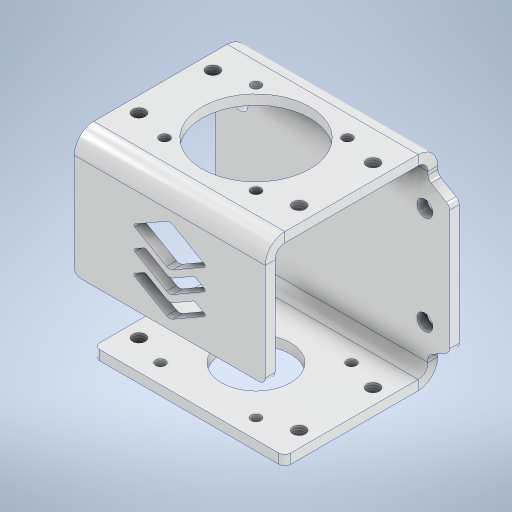
# Autodesk Inventor part: Z-Axis Drive Mount
Saved by Autodesk Inventor 2024 (Build 280153000, 153)
## iProperties
Created: 2024-12-16
Part Number: Z-Axis Drive Mount
Material: Aluminum 6061
Document SubType Name: Sheet Metal
Designer: Ishaan
Density: 2.7 g/cm^3
Sheet Metal Rule: SendCutSend_1-8_Alu
Appearance: Aluminum - Flat
Flat Pattern Width: 7.6 cm
Flat Pattern Length: 19.5495 cm
Flat Pattern Area: 148.576 cm^2
Sheet Metal Width: 76.000 mm
Sheet Metal Length: 195.495 mm
Sheet Metal Area: 14857.623 mm^2
Author: Ishaan
Autodesk Inventor part; units mm, degrees
note: some values were not read from the file. Chosen so that the rebuilt part matches the saved one: direction of "Hole1"; direction of "Hole2"; direction of "Hole3"; direction of "Hole4".
ref_plane "YZ Plane" through (0, 0, 0) normal (1, 0, 0) x (0, 1, 0)
ref_plane "XZ Plane" through (0, 0, 0) normal (0, 1, 0) x (-1, 0, 0)
ref_plane "XY Plane" through (0, 0, 0) normal (0, 0, 1) x (1, 0, 0)
sketch "Sketch1" plane through (0, 0, 0) normal (0, 0, 1) x (1, 0, 0)
  line L0 (31, -30.025) -> (-31, -30.025)
  line L1 (-31, -30.025) -> (-31, 30.025)
  line L2 (-31, 30.025) -> (31, 30.025)
  line L3 (31, 30.025) -> (31, -30.025)
  line L4 (31, -30.025) -> (-31, 30.025) construction
  line L5 (-31, -30.025) -> (31, 30.025) construction
  point P0 (0, 0)
  dimension "d0" = 62
  dimension "d1" = 60.05
  measures "d0" distance of L1.end L2.end
  measures "d1" distance of L0.end L1.end
extrude "Plate1" add sketch "Sketch1" along normal blind 3.175
sketch "Sketch2" plane through (-31, 30.025, 3.175) normal (0, 1, 0) x (-1, 0, 0)
  line L0 (-62, 0) -> (0, 0)
  line L1 (0, 0) -> (0, 71.825)
  line L2 (0, 71.825) -> (-62, 71.825)
  line L3 (-62, 71.825) -> (-62, 0)
  constraints: 6 end point, 1 horizontal, 1 perpendicular, 1 vertical
edge flange "Flange1" height 75 angle 90 thickness 3.175 bend radius 3.175 thickness toward (0, 1, 0) relief tear relief width 3.175 relief depth 1.5875 edges at (0, 30.025, 3.175) wall of the first edge with corners at (31, 30.025, 3.175) (-31, 30.025, 3.175) (-31, 30.025, 75) (31, 30.025, 75)
bend "Bend1"
corner "Corner1"
sketch "Sketch3" plane through (31, -30.025, 3.175) normal (0, -1, 0) x (1, 0, 0)
  line L0 (-62, 0) -> (0, 0)
  line L1 (0, 0) -> (0, 71.825)
  line L2 (0, 71.825) -> (-62, 71.825)
  line L3 (-62, 71.825) -> (-62, 0)
  constraints: 6 end point, 1 horizontal, 1 perpendicular, 1 vertical
edge flange "Flange2" height 75 angle 90 thickness 3.175 bend radius 3.175 thickness toward (0, -1, 0) relief tear relief width 3.175 relief depth 1.5875 edges at (0, -30.025, 3.175) wall of the first edge with corners at (-31, -30.025, 3.175) (31, -30.025, 3.175) (31, -30.025, 75) (-31, -30.025, 75)
bend "Bend2"
corner "Corner2"
sketch "Sketch4" plane through (-31, 33.2, 75) normal (0, 1, 0) x (1, 0, 0)
  line L0 (52, 26) -> (10, 26) construction
  line L1 (10, 26) -> (10, 68) construction
  line L2 (10, 68) -> (52, 68) construction
  line L3 (52, 68) -> (52, 26) construction
  line L4 (52, 26) -> (10, 68) construction
  line L5 (10, 26) -> (52, 68) construction
  circle A0 centre (31, 47) radius 21 construction
  line L6 (0, 0) -> (0, 68.65) projected
  line L7 (0, 25.35) -> (62, 25.35)
  line L8 (62, 68.65) -> (0, 68.65) projected
  line L9 (0, 0) -> (0, 68.65) projected
  line L10 (62, 0) -> (0, 0) projected
  line L11 (62, 68.65) -> (62, 0) projected
  line L12 (62, 68.65) -> (62, 0) projected
  circle A1 centre (31, 47) radius 17.5
  line L13 (57, 35) -> (5, 35)
  line L14 (5, 35) -> (5, 59)
  line L15 (5, 59) -> (57, 59)
  line L16 (57, 59) -> (57, 35)
  line L17 (57, 35) -> (5, 59) construction
  line L18 (5, 35) -> (57, 59) construction
  point P0 (31, 75)
  point P1 (16.1508, 61.8492)
  point P2 (45.8492, 61.8492)
  point P3 (45.8492, 32.1508)
  point P4 (16.1508, 32.1508)
  point P5 (62, 25.35)
  point P6 (31, 47)
  dimension "d23" = 42
  dimension "d24" = 42
  dimension "d25" = 28
  dimension "d26" = 42
  dimension "d32" = 35
  dimension "d75" = 24
  dimension "d76" = 5
  dimension "d77" = 0
  dimension "d78" = 9.65
  dimension "d99" = 5
  dimension "d127" = 21.65
  dimension "d128" = 21.65
  constraints: 26 end point, 7 coincident, 6 point on line, 4 midpoint, 4 parallel, 4 point on circle, 3 horizontal, 2 centre point, 2 perpendicular, 1 vertical alignment
  measures "d23" distance of L1.end L2.end
  measures "d24" distance of L0.end L1.end
  measures "d25" distance of point (31, 75) point (31, 47)
  measures "d26" diameter of A0
  measures "d32" diameter of A1
  measures "d75" distance of L13.end L14.end
  measures "d76" distance between parallel lines of L6 L14
  measures "d77" distance of A1.centre point (31, 47)
  measures "d78" distance from line of L7 L13.end
  measures "d99" distance between parallel lines of L14 L1
  measures "d127" distance from line of A0.centre L7
  measures "d128" distance from line of L8 point (31, 47)
extrude "Extrusion1" cut sketch "Sketch4" against normal up to surface (3.175 mm away) contours L6 L7 L11 L10
extrude "Extrusion2" cut sketch "Sketch4" against normal up to surface (3.175 mm away) contours A1 L13 L15 | L15 A1 | A1 L13
hole "Hole1" at (-14.8492, 33.2, 13.1508) at (14.8492, 33.2, 13.1508) at (14.8492, 33.2, 42.8492) at (-14.8492, 33.2, 42.8492) direction (0, -1, 0) diameter 3.242 depth 3.175 thread size "M4x0.7" class "6H" standard "ANSI Metric M Profile"
hole "Hole2" at (-26, 33.2, 40) at (-26, 33.2, 16) at (26, 33.2, 40) at (26, 33.2, 16) direction (0, -1, 0) diameter 4.134 depth 3.175 thread size "M5x0.8" class "6H" standard "ANSI Metric M Profile"
sketch "Sketch5" plane through (-31, -33.2, 75) normal (0, -1, 0) x (1, 0, 0)
  circle A0 centre (31, -47) radius 17.5 construction
  circle A1 centre (31, -47) radius 11.25
  line L0 (46.5, -62.5) -> (15.5, -62.5) construction
  line L1 (15.5, -62.5) -> (15.5, -31.5) construction
  line L2 (15.5, -31.5) -> (46.5, -31.5) construction
  line L3 (46.5, -31.5) -> (46.5, -62.5) construction
  line L4 (46.5, -62.5) -> (15.5, -31.5) construction
  line L5 (15.5, -62.5) -> (46.5, -31.5) construction
  line L6 (0, -68.65) -> (62, -68.65) projected
  line L7 (62, 0) -> (62, -68.65) projected
  line L8 (0, 0) -> (62, 0) projected
  line L9 (0, -68.65) -> (0, 0) projected
  line L10 (0, -25.35) -> (62, -25.35)
  circle A2 centre (5, -59) radius 2.067 projected
  circle A3 centre (5, -35) radius 2.067 projected
  circle A4 centre (57, -35) radius 2.067 projected
  circle A5 centre (57, -59) radius 2.067 projected
  point P0 (31, -75)
  dimension "d49" = 22.5
  dimension "d50" = 31
  dimension "d51" = 31
  dimension "d52" = 5
  dimension "d53" = 9.65
  dimension "d65" = 21.65
  constraints: 14 end point, 13 coincident, 2 midpoint, 2 parallel, 2 perpendicular, 2 point on line, 1 centre point, 1 horizontal
  measures "d49" diameter of A1
  measures "d50" distance of L1.end L2.end
  measures "d51" distance of L0.end L1.end
  measures "d52" distance from line of L7 point (57, -35)
  measures "d53" distance from line of L10 point (57, -35)
  measures "d65" distance from line of L10 A0.centre
extrude "Extrusion3" cut sketch "Sketch5" against normal blind 3.175 contours L9 L8 L7 L10
extrude "Extrusion4" cut sketch "Sketch5" against normal up to surface (3.175 mm away) contours A1
hole "Hole3" at (15.5, -33.2, 43.5) at (-15.5, -33.2, 43.5) at (15.5, -33.2, 43.5) at (15.5, -33.2, 12.5) at (-15.5, -33.2, 12.5) direction (0, 1, 0) diameter 3.2 depth 3.175
hole "Hole4" at (-26, -33.2, 16) at (26, -33.2, 16) at (26, -33.2, 40) at (-26, -33.2, 40) direction (0, 1, 0) diameter 4.134 depth 3.175 thread size "M5x0.8" class "6H" standard "ANSI Metric M Profile"
sketch "Sketch8" plane through (0, 0, 3.175) normal (0, 0, 1) x (1, 0, 0)
  line L0 (30, -16) -> (-30, -16)
  line L1 (-30, -16) -> (-30, 16)
  line L2 (-30, 16) -> (30, 16)
  line L3 (30, 16) -> (30, -16)
  line L4 (30, -16) -> (-30, 16) construction
  line L5 (-30, -16) -> (30, 16) construction
  line L6 (-30, 25.2376) -> (-22, 20.6188)
  line L7 (-22, 20.6188) -> (-22, 11.3812)
  line L8 (-22, 11.3812) -> (-30, 6.7624)
  line L9 (-30, 6.7624) -> (-38, 11.3812)
  line L10 (-38, 11.3812) -> (-38, 20.6188)
  line L11 (-38, 20.6188) -> (-30, 25.2376)
  line L12 (-30, -25.2376) -> (-38, -20.6188)
  line L13 (-38, -20.6188) -> (-38, -11.3812)
  line L14 (-38, -11.3812) -> (-30, -6.7624)
  line L15 (-30, -6.7624) -> (-22, -11.3812)
  line L16 (-22, -11.3812) -> (-22, -20.6188)
  line L17 (-22, -20.6188) -> (-30, -25.2376)
  line L18 (-38, 11.3812) -> (-38, -11.3812)
  circle A0 centre (-30, 16) radius 8 construction
  point P0 (0, 0)
  point P1 (-22, -16)
  point P2 (-22, 16)
  dimension "d100" = 60
  dimension "d101" = 32
  dimension "d102" = 8
  dimension "d103" = 16
  dimension "d115" = 38
  constraints: 38 end point, 7 coincident, 3 vertical, 2 midpoint, 2 parallel, 1 centre point, 1 horizontal, 1 perpendicular, 1 tangent, 26 other
  measures "d100" distance of L1.end L2.end
  measures "d101" distance of L0.end L1.end
  measures "d102" distance between parallel lines of L18 L1
  measures "d103" diameter of A0
  measures "d115" distance from line of point (0, 0) L18
extrude "Extrusion5" add sketch "Sketch8" against normal up to surface (3.175 mm away) contours L16 L17 L12 L13 L14 L1 L0 | L2 L1 L9 L10 L11 L6 L7 | L14 L18 L9 L1
mirror "Mirror1" about plane through (0, 0, 0) normal (1, 0, 0) of "Extrusion5"
fillet "Fillet3" radius 2 8 edges at (-31, -24.6603, 1.5875) (-38, -20.6188, 1.5875) (-38, 20.6188, 1.5875) (-31, 24.6603, 1.5875) (31, 24.6603, 1.5875) (38, 20.6188, 1.5875) (31, -24.6603, 1.5875) (38, -20.6188, 1.5875)
hole "Hole6" at (-30, 16, 3.175) at (-30, -16, 3.175) at (30, -16, 3.175) at (30, 16, 3.175) direction (0, 0, -1) diameter 5.2 end through all
fillet "Fillet1" radius 2 2 edges at (31, -31.6125, 49.65) (-31, -31.6125, 49.65)
sketch "Sketch7" plane through (-31, 26.85, 52.825) normal (0, 0, 1) x (1, 0, 0)
  line L0 (62, 0) -> (0, 0)
  line L1 (0, 0) -> (0, -33.65)
  line L2 (0, -33.65) -> (62, -33.65)
  line L3 (62, -33.65) -> (62, 0)
  constraints: 6 end point, 1 horizontal, 1 perpendicular, 1 vertical
edge flange "Flange3" height 40 angle 90 thickness 3.175 bend radius 3.175 thickness toward (0, 0, 1) relief tear relief width 3.175 relief depth 1.5875 edges at (0, 30.025, 49.65) wall of the first edge with corners at (31, 26.85, 52.825) (-31, 26.85, 52.825) (-31, -6.8, 52.825) (31, -6.8, 52.825)
bend "Bend3"
corner "Corner3"
sketch "Sketch9" plane through (-31, -6.8, 56) normal (0, 0, 1) x (1, 0, 0)
  line L0 (62, 33.65) -> (0, 33.65) construction
  line L1 (0, 0) -> (0, 33.65) construction
  line L2 (62, 0) -> (0, 0) construction
  line L3 (62, 33.65) -> (62, 0) construction
  line L4 (19, 23.7532) -> (31, 30.6814)
  line L5 (31, 30.6814) -> (43, 23.7532)
  line L6 (43, 23.7532) -> (43, 9.8968)
  line L7 (43, 9.8968) -> (31, 2.9686)
  line L8 (31, 2.9686) -> (19, 9.8968)
  line L9 (19, 9.8968) -> (19, 23.7532)
  line L10 (31, 16.825) -> (43, 23.7532)
  line L11 (31, 16.825) -> (19, 23.7532)
  line L12 (19, 21.4438) -> (31, 14.5156)
  line L13 (31, 14.5156) -> (43, 21.4438)
  line L14 (19, 16.825) -> (31, 9.8968)
  line L15 (31, 9.8968) -> (43, 16.825)
  line L16 (43, 14.5156) -> (31, 7.5874)
  line L17 (31, 7.5874) -> (19, 14.5156)
  line L18 (19, 16.825) -> (23, 19.1344)
  line L19 (43, 16.825) -> (39, 19.1344)
  line L20 (43, 9.8968) -> (39, 12.2062)
  line L21 (19, 9.8968) -> (23, 12.2062)
  point P0 (31, 6.8)
  point P1 (0, 16.825)
  dimension "d116" = 2
  dimension "d117" = 4
  dimension "d118" = 2
  dimension "d119" = 4
  dimension "d120" = 24
  constraints: 36 end point, 10 parallel, 8 point on line, 5 vertical alignment, 3 midpoint, 1 horizontal alignment, 1 vertical, 13 other
  measures "d116" distance between parallel lines of L11 L12
  measures "d117" distance between parallel lines of L12 L14
  measures "d118" distance between parallel lines of L17 L14
  measures "d119" distance between parallel lines of L8 L17
  measures "d120" distance between parallel lines of L6 L9
extrude "Extrusion6" cut sketch "Sketch9" against normal up to surface (3.175 mm away) contours L4 L5 L10 L11 | L18 L12 L13 L19 L15 L14 | L21 L17 L16 L20 L7 L8
fillet "Fillet4" radius 2 6 edges at (0, 23.8814, 54.4125) (0, 10.025, 54.4125) (0, 7.7156, 54.4125) (0, 3.0968, 54.4125) (0, 0.7874, 54.4125) (0, -3.8314, 54.4125)
fillet "Fillet5" radius 0.5 6 edges at (-12, 16.9532, 54.4125) (-12, 10.025, 54.4125) (-12, 3.0968, 54.4125) (12, 3.0968, 54.4125) (12, 10.025, 54.4125) (12, 16.9532, 54.4125)
fillet "Fillet6" radius 1 4 edges at (-8, 5.4062, 54.4125) (-8, 12.3344, 54.4125) (8, 12.3344, 54.4125) (8, 5.4062, 54.4125)
fillet "Fillet7" radius 2 2 edges at (31, -6.8, 54.4125) (-31, -6.8, 54.4125)
equation "\"d76\" = d99"
equation "\"d127\" = d128"
equation "\"d40\" = Thickness"
equation "\"d47\" = d27"
equation "\"d117\" = 2 * d116"
equation "\"d118\" = d116"
equation "\"d119\" = d117"
equation "\"d2\" = Thickness"
equation "\"d3\" = BendReliefWidth"
equation "\"d4\" = BendReliefDepth"
equation "\"d5\" = MinimumRemnant"
equation "\"d6\" = TransitionRadius"
equation "\"d9\" = BendRadius"
equation "\"d10\" = CornerReliefSize"
equation "\"d11\" = GapSize"
equation "\"d12\" = JacobiRadiusSize"
equation "\"d13\" = BendReliefWidth"
equation "\"d14\" = BendReliefDepth"
equation "\"d15\" = MinimumRemnant"
equation "\"d16\" = TransitionRadius"
equation "\"d19\" = BendRadius"
equation "\"d20\" = CornerReliefSize"
equation "\"d21\" = GapSize"
equation "\"d22\" = JacobiRadiusSize"
equation "\"d89\" = BendReliefWidth"
equation "\"d90\" = BendReliefDepth"
equation "\"d91\" = MinimumRemnant"
equation "\"d92\" = TransitionRadius"
equation "\"d95\" = BendRadius"
equation "\"d96\" = CornerReliefSize"
equation "\"d97\" = GapSize"
equation "\"d98\" = JacobiRadiusSize"
equation "\"BendReliefWidth\" = Thickness"
equation "\"BendReliefDepth\" = 0.5 * Thickness"
equation "\"CornerReliefSize\" = 4 * Thickness"
equation "\"MinimumRemnant\" = 2 * Thickness"
equation "\"TransitionRadius\" = BendRadius"
equation "\"JacobiRadiusSize\" = BendRadius"
equation "\"GapSize\" = Thickness"
equation "\"Thickness\" = 3.175"
equation "\"d27\" = 24"
equation "\"BendRadius\" = 3.175"
body "Solid1"
